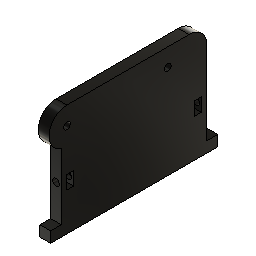
AsseblyCameraHead v2 (Autodesk Fusion 360 archive; units mm, degrees)
design "CameraHeadHolder"
Autodesk Fusion 360 part; units mm, degrees
sketch "Sketch1" plane through (0, 0, 0) normal (1, 0, 0) x (0, 1, 0)
  line L0 (-32.5, 4.8) -> (-37.3, 4.8)
  line L1 (-37.3, 4.8) -> (-37.3, 0)
  line L2 (-37.3, 0) -> (37.3, 0)
  line L3 (37.3, 0) -> (37.3, 4.8)
  line L4 (37.3, 4.8) -> (32.5, 4.8)
  line L5 (-32.5, 4.8) -> (-32.5, 34.2007)
  line L6 (-30, 49.8) -> (24.5, 49.8)
  line L7 (32.5, 41.8) -> (32.5, 4.8)
  line L8 (-30, 41.8) -> (15, 41.8) construction
  circle A0 centre (-30, 41.8) radius 1.5
  line L9 (15, 41.8) -> (24.5, 41.8) construction
  arc A1 (24.5, 49.8) -> (32.5, 41.8) centre (24.5, 41.8) ccw construction
  arc A2 (32.5, 41.8) -> (24.5, 49.8) centre (24.5, 41.8) ccw
  line L10 (24.5, 49.8) -> (32.5, 49.8) construction
  line L11 (32.5, 49.8) -> (32.5, 41.8) construction
  circle A3 centre (15, 41.8) radius 1.5
  circle A4 centre (-25, 41.8) radius 5 construction
  circle A5 centre (25, 41.8) radius 5 construction
  line L12 (-25, 41.8) -> (25, 41.8) construction
  line L13 (0, 41.8) -> (0, 0) construction
  arc A6 (-32.5, 34.2007) -> (-30, 49.8) centre (-30, 41.8) ccw construction
  arc A7 (-30, 49.8) -> (-32.5, 34.2007) centre (-30, 41.8) ccw
  point P0 (0, 41.8)
  dimension "d1" = 4.8
  dimension "d2" = 4.8
  dimension "d3" = 74.6
  dimension "d4" = 4.8
  dimension "d5" = 4.8
  dimension "d6" = 45
  dimension "d8" = 45
  dimension "d9" = 8
  dimension "d11" = 3
  dimension "d12" = 16
  dimension "d13" = 3
  dimension "d14" = 10
  dimension "d15" = 10
  dimension "d16" = 50
  dimension "d17" = 10
  constraint horizontal L0
  constraint perpendicular L0 L1
  constraint perpendicular L1 L2
  constraint perpendicular L2 L3
  constraint perpendicular L3 L4
  constraint midpoint L2 L13.end
  constraint coincident L13.end origin
  constraint perpendicular L0 L5
  constraint perpendicular L5 L6
  constraint perpendicular L4 L7
  constraint perpendicular L7 L8
  constraint tangent L7 A1
  constraint coincident L9.end A1.centre
  constraint parallel L8 L9
  constraint concentric A1 A2
  constraint perpendicular L5 L10
  constraint perpendicular L4 L11
  constraint coincident L8.end L9.start
  constraint coincident L8 A4.centre
  constraint coincident L9 A5.centre
  constraint coincident A4.centre L12.start
  constraint coincident A5.centre L12.end
  constraint midpoint L12 P0
  constraint coincident P0 L13.start
  constraint vertical L13
  constraint coincident L8.start A0.centre
  constraint tangent L6 A6
  constraint concentric A6 A7
  constraint concentric A0 A7
  measures "d1" distance of L0.start L0.end
  measures "d2" distance of L0.end L1.end
  measures "d3" distance of L1.end L2.end
  measures "d4" distance of L2.end L3.end
  measures "d5" distance of L3.end L4.end
  measures "d6" distance of L4 L6
  measures "d8" distance of L8.start L8.end
  measures "d9" distance of L6 L8
  measures "d11" diameter of A0
  measures "d12" diameter of A1
  measures "d13" diameter of A3
  measures "d14" diameter of A4
  measures "d15" diameter of A5 L6
  measures "d16" distance of A4.centre A5.centre
  measures "d17" distance of L8.end A5.centre
extrude "Extrude1" add sketch "Sketch1" along normal blind 4.8
sketch "Sketch2" plane through (0, -32.5, 0) normal (0, -1, 0) x (1, 0, 0)
  line L0 (0, 34.2007) -> (0, 4.8)
  line L1 (0, 4.8) -> (4.8, 4.8)
  line L2 (4.8, 4.8) -> (4.8, 34.2007)
  line L3 (4.8, 34.2007) -> (0, 34.2007)
  line L4 (0, 4.8) -> (0, 0)
  line L5 (0, 0) -> (4.8, 0)
  line L6 (4.8, 0) -> (4.8, 4.8)
  line L7 (4.8, 4.8) -> (0, 4.8)
  circle A0 centre (2.4, 20) radius 1.5
  dimension "d20" = 3
  dimension "d21" = 20
  dimension "d22" = 2.4
  measures "d20" diameter of A0
  measures "d21" distance of L5 A0.centre
  measures "d22" distance of L2 A0.centre
hole "Hole1" at (2.4, -32.5, 20) direction (0, 1, 0) diameter 3 depth 7.2 tip angle 118
sketch "Sketch3" plane through (0, 32.5, 0) normal (0, 1, 0) x (-1, 0, 0)
  line L0 (0, 4.8) -> (0, 41.8)
  line L1 (0, 41.8) -> (-4.8, 41.8)
  line L2 (-4.8, 41.8) -> (-4.8, 4.8)
  line L3 (-4.8, 4.8) -> (0, 4.8)
  line L4 (0, 0) -> (0, 4.8)
  line L5 (0, 4.8) -> (-4.8, 4.8)
  line L6 (-4.8, 4.8) -> (-4.8, 0)
  line L7 (-4.8, 0) -> (0, 0)
  circle A0 centre (-2.4, 20) radius 1.5
  dimension "d26" = 3
  dimension "d27" = 20
  dimension "d28" = 2.4
  measures "d26" diameter of A0
  measures "d27" distance of L7 A0.centre
  measures "d28" distance of L0 A0.centre
hole "Hole2" at (2.4, 32.5, 20) direction (0, -1, 0) diameter 3 depth 7.2 tip angle 118
sketch "Sketch4" plane through (4.8, 0, 0) normal (1, 0, 0) x (0, 1, 0)
  circle A0 centre (15, 41.8) radius 1.5
  circle A1 centre (-30, 41.8) radius 1.5
  arc A2 (32.5, 41.8) -> (24.5, 49.8) centre (24.5, 41.8) ccw
  line L0 (24.5, 49.8) -> (-30, 49.8)
  arc A3 (-30, 49.8) -> (-32.5, 34.2007) centre (-30, 41.8) ccw
  line L1 (-32.5, 34.2007) -> (-32.5, 4.8)
  line L2 (-32.5, 4.8) -> (-37.3, 4.8)
  line L3 (-37.3, 4.8) -> (-37.3, 0)
  line L4 (-37.3, 0) -> (37.3, 0)
  line L5 (37.3, 0) -> (37.3, 4.8)
  line L6 (37.3, 4.8) -> (32.5, 4.8)
  line L7 (32.5, 4.8) -> (32.5, 41.8)
  line L8 (-32.5, 18.5) -> (-25.3, 18.5) construction
  line L9 (-25.3, 18.5) -> (-25.3, 21.5) construction
  line L10 (-25.3, 21.5) -> (-32.5, 21.5) construction
  line L11 (32.5, 21.5) -> (25.3, 21.5) construction
  line L12 (25.3, 21.5) -> (25.3, 18.5) construction
  line L13 (25.3, 18.5) -> (32.5, 18.5) construction
  line L14 (-25.3, 20) -> (25.3, 20) construction
  line L15 (-30, 17) -> (-27, 17)
  line L16 (-27, 17) -> (-27, 23)
  line L17 (-27, 23) -> (-30, 23)
  line L18 (-30, 23) -> (-30, 17)
  line L19 (-25.3, 20) -> (-27, 20) construction
  line L20 (27, 23) -> (30, 23)
  line L21 (30, 23) -> (30, 17)
  line L22 (30, 17) -> (27, 17)
  line L23 (27, 17) -> (27, 23)
  line L24 (27, 20) -> (25.3, 20) construction
  point P0 (-25.3, 20)
  point P1 (25.3, 20)
  point P2 (-27, 20)
  point P3 (27, 20)
  dimension "d32" = 7.2
  dimension "d33" = 3
  dimension "d34" = 7.2
  dimension "d35" = 3
  dimension "d36" = 20
  dimension "d37" = 3
  dimension "d38" = 6
  dimension "d39" = 2.5
  dimension "d40" = 3
  dimension "d41" = 6
  dimension "d42" = 2.5
  constraint coincident L1 L8.start
  constraint perpendicular L1 L8
  constraint perpendicular L8 L9
  constraint coincident L1 L10.end
  constraint perpendicular L1 L10
  constraint midpoint L9 P0
  constraint coincident L7 L11.start
  constraint perpendicular L7 L11
  constraint perpendicular L11 L12
  constraint coincident L7 L13.end
  constraint perpendicular L7 L13
  constraint midpoint L12 P1
  constraint coincident P0 L14.start
  constraint coincident P1 L14.end
  constraint horizontal L14
  constraint horizontal L15
  constraint vertical L16
  constraint horizontal L17
  constraint vertical L18
  constraint midpoint L16 P2
  constraint coincident P2 L19.end
  constraint horizontal L19
  constraint horizontal L20
  constraint vertical L21
  constraint horizontal L22
  constraint vertical L23
  constraint midpoint L23 P3
  constraint coincident P3 L24.start
  constraint horizontal L24
  measures "d32" distance of L8.start L8.end
  measures "d33" distance of L8.end L9.end
  measures "d34" distance of L11.start L11.end
  measures "d35" distance of L11.end L12.end
  measures "d36" distance of L4 L14
  measures "d37" distance of L15.start L15.end
  measures "d38" distance of L15.start L17.end
  measures "d39" distance of L1 L18
  measures "d40" distance of L20.start L20.end
  measures "d41" distance of L20.start L22.end
  measures "d42" distance of L7 L21
extrude "Extrude2" cut sketch "Sketch4" against normal through all contours L15 L16 L17 L18 | L20 L21 L22 L23
